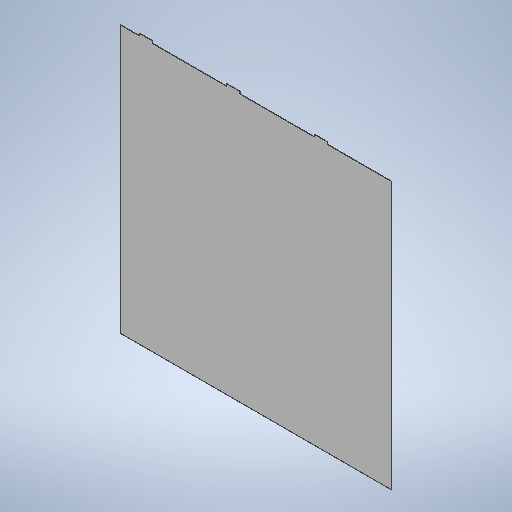
# Autodesk Inventor part: Heat sheild
Saved by Autodesk Inventor 2025.1 (Build 291241020, 241B)
## iProperties
Created: 2024-09-24
Part Number: Heat sheild
Material: Generic
Document SubType Name: Modeling
Designer: jjk
Density: 1 g/cm^3
Appearance: Default
Author: jjk
Autodesk Inventor part; units mm, degrees
ref_plane "YZ Plane" through (0, 0, 0) normal (1, 0, 0) x (0, 1, 0)
ref_plane "XZ Plane" through (0, 0, 0) normal (0, 1, 0) x (-1, 0, 0)
ref_plane "XY Plane" through (0, 0, 0) normal (0, 0, 1) x (1, 0, 0)
sketch "Sketch1" plane through (0, 0, 0) normal (0, 0, 1) x (1, 0, 0)
  line L0 (0, 0) -> (157.48, 0)
  line L1 (157.48, 0) -> (157.48, 154.94)
  line L2 (0, 154.94) -> (0, 0)
  line L3 (18.6436, 154.94) -> (18.6436, 156.21)
  line L4 (18.6436, 156.21) -> (11.0236, 156.21)
  line L5 (11.0236, 156.21) -> (11.0236, 154.94)
  line L6 (61.8236, 154.94) -> (61.8236, 156.21)
  line L7 (61.8236, 156.21) -> (69.4436, 156.21)
  line L8 (69.4436, 156.21) -> (69.4436, 154.94)
  line L9 (120.2436, 154.94) -> (120.2436, 156.21)
  line L10 (120.2436, 156.21) -> (112.6236, 156.21)
  line L11 (112.6236, 156.21) -> (112.6236, 154.94)
  line L12 (61.8236, 154.94) -> (18.6436, 154.94)
  line L13 (11.0236, 154.94) -> (0, 154.94)
  line L14 (157.48, 154.94) -> (120.2436, 154.94)
  line L15 (112.6236, 154.94) -> (69.4436, 154.94)
  dimension "d0" = 154.94
  dimension "d1" = 157.48
  dimension "d4" = 7.62
  dimension "d8" = 7.62
  dimension "d10" = 112.6236
  dimension "d11" = 1.27
  dimension "d12" = 11.0236
  dimension "d13" = 1.27
  dimension "d14" = 7.62
  dimension "d15" = 7.62
  dimension "d16" = 1.27
  constraints: 32 end point, 8 parallel, 1 horizontal, 1 perpendicular
  measures "d0" distance of L0.end L1.end
  measures "d1" distance of L0.start L0.end
  measures "d4" distance of L3.end L4.end
  measures "d8" distance of L9.end L10.end
  measures "d10" distance between parallel lines of L2 L11
  measures "d11" distance between parallel lines of L12 L4
  measures "d12" distance between parallel lines of L2 L5
  measures "d13" distance between parallel lines of L12 L7
  measures "d14" distance of L6.end L7.end
  measures "d15" distance between parallel lines of L8 L6
  measures "d16" distance between parallel lines of L15 L10
extrude "Extrusion1" add sketch "Sketch1" along normal blind 0.254
body "Solid1"
